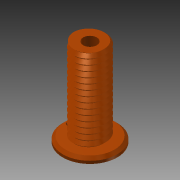
# Autodesk Inventor part: z pulley
Saved by Autodesk Inventor 2013 (Build 170138000, 138)
## iProperties
Created: 2013-09-18
Part Number: z pulley
Material: Generic
Document SubType Name: Modeling
Designer: employee
Density: 1 g/cm^3
Mass: 2.82224 g
Surface Area: 26.5069 cm^2
Volume: 2.82224 cm^3
Author: employee
Autodesk Inventor part; units mm, degrees
ref_plane "YZ Plane" through (0, 0, 0) normal (1, 0, 0) x (0, 1, 0)
ref_plane "XZ Plane" through (0, 0, 0) normal (0, 1, 0) x (-1, 0, 0)
ref_plane "XY Plane" through (0, 0, 0) normal (0, 0, 1) x (1, 0, 0)
sketch "Sketch1" plane through (0, 0, 0) normal (0, 0, 1) x (1, 0, 0)
  circle A0 centre (0, 0) radius 5
  dimension "d0" = 10
  constraints: 1 centre point, 1 coincident
  measures "d0" diameter of A0
extrude "Extrusion1" add sketch "Sketch1" along normal blind 30
sketch "Sketch2" plane through (0, 0, 0) normal (0, 0, -1) x (-1, 0, 0)
  circle A0 centre (0, 0) radius 5 projected
  circle A1 centre (0, 0) radius 10
  dimension "d28" = 20
  constraints: 1 centre point, 1 coincident
  measures "d28" diameter of A1
extrude "Extrusion2" add sketch "Sketch2" along normal blind 2 contours A0 | A1
sketch "Sketch3" plane through (0, 0, 0) normal (0, 1, 0) x (-1, 0, 0)
  line L0 (5, 0) -> (10, 0) projected
  line L1 (10, 0) -> (10, -2) projected
  line L2 (10, -2) -> (-10, -2) projected
  line L3 (-10, -2) -> (-10, 0) projected
  line L4 (-10, 0) -> (-5, 0) projected
  line L5 (-5, 0) -> (-5, 30) projected
  line L6 (-5, 30) -> (5, 30) projected
  line L7 (5, 30) -> (5, 0) projected
  line L8 (-5, 30) -> (-5, 32)
  line L9 (-5, 32) -> (-6, 31)
  line L10 (-6, 31) -> (-5, 30)
  point P0 (0, 0)
  dimension "d7" = 2
  constraints: 6 end point, 2 perpendicular, 1 parallel
  measures "d7" distance of L5.end L8.end
coil "Coil1" sketch "Sketch3" operation add axis through (0, 0, -10) along (0, 0, -1) pitch 2.001 turns 16 hand right contours L10 L9 L8
sketch "Sketch8" plane through (0, 0, -2) normal (0, 0, -1) x (-1, 0, 0)
  circle A0 centre (0, 0) radius 10 projected
extrude "Extrusion7" cut sketch "Sketch8" along normal blind 10
chamfer "Chamfer1" distance 1 angle 45 1 edges at (10, 0, 0)
sketch "Sketch4" plane through (0, 0, 30) normal (0, 0, 1) x (1, 0, 0)
  arc A0 (5, 0.0157) -> (5, 0) centre (0, 0) ccw projected
  circle A1 centre (0, 0) radius 20
  dimension "d19" = 40
  constraints: 1 centre point, 1 coincident
  measures "d19" diameter of A1
extrude "Extrusion3" cut sketch "Sketch4" along normal through all
sketch "Sketch5" plane through (0, 0, 30) normal (0, 0, 1) x (1, 0, 0)
  arc A0 (5, 0) -> (5, 0.0157) centre (0, 0) ccw projected
  circle A1 centre (0, 0) radius 2.5
  dimension "d23" = 5
  constraints: 1 centre point, 1 coincident
  measures "d23" diameter of A1
extrude "Extrusion4" cut sketch "Sketch5" against normal through all
sketch "Sketch6" plane through (0, 0, 0) normal (0, 0, 1) x (1, 0, 0)
  circle A0 centre (0, 0) radius 9 projected
  circle A1 centre (-7.4931, 0) radius 1
  circle A2 centre (-7.4931, 0) radius 1.5069
  dimension "d47" = 2
  constraints: 2 centre point, 1 coincident, 1 horizontal alignment, 1 tangent, 2 other
  measures "d47" diameter of A1
extrude "Extrusion8" cut sketch "Sketch6" against normal through all contours A1
body "Solid1"
